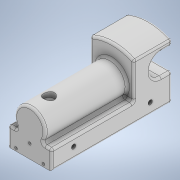
# Autodesk Inventor part: DERKS Train Body
Saved by Autodesk Inventor 2020 (Build 240168000, 168)
## iProperties
Created: 2020-04-30
Part Number: DERKS Train Body
Material: Generic
Document SubType Name: Modeling
Designer: tader
Density: 1 g/cm^3
Appearance: Default
Author: tader
Autodesk Inventor part; units mm, degrees
ref_plane "YZ Plane" through (0, 0, 0) normal (1, 0, 0) x (0, 1, 0)
ref_plane "XZ Plane" through (0, 0, 0) normal (0, 1, 0) x (-1, 0, 0)
ref_plane "XY Plane" through (0, 0, 0) normal (0, 0, 1) x (1, 0, 0)
sketch "Sketch3" plane through (0, 0, 0) normal (1, 0, 0) x (0, 1, 0)
  line L0 (10.0868, 77.2075) -> (-12.1382, 77.2075)
  line L1 (-12.1382, 77.2075) -> (-12.1382, -62.4925)
  line L2 (-12.1382, -62.4925) -> (76.5771, -62.4925)
  line L3 (76.5771, -62.4925) -> (76.5771, -18.0425)
  line L4 (76.5771, -18.0425) -> (10.0868, -18.0425)
  line L5 (10.0868, -18.0425) -> (10.0868, 77.2075)
  point P0 (0, 0)
  dimension "d1" = 22.225
  dimension "d2" = 139.7
  dimension "d3" = 44.45
  constraints: 12 end point, 4 perpendicular, 1 horizontal, 1 vertical
  measures "d1" distance of L0.start L0.end
  measures "d2" distance of L0.end L1.end
  measures "d3" distance of L2.end L3.end
extrude "Extrusion1" add sketch "Sketch3" along normal blind 50.8
sketch "Sketch4" plane through (0, -12.1382, 77.2075) normal (0, 0, 1) x (1, 0, 0)
  line L0 (0, 0) -> (50.8, 0) projected
  line L1 (25.4, 0) -> (25.4, 34.925)
  line L2 (0, 22.225) -> (50.8, 22.225) projected
  arc A0 (37.9356, 22.225) -> (12.8644, 22.225) centre (25.4, 34.925) ccw
  point P0 (0, 12.1382)
  dimension "d6" = 34.925
  constraints: 2 end point, 2 point on circle, 2 point on line, 1 centre point, 1 coincident, 1 midpoint, 1 vertical
  measures "d6" distance of L1.start L1.end
extrude "Extrusion2" add sketch "Sketch4" against normal up to surface (139.7 mm away)
sketch "Sketch5" plane through (50.8, 0, 0) normal (1, 0, 0) x (0, 0, -1)
  line L0 (18.0425, 76.5771) -> (18.0425, 10.0868) projected
  line L1 (18.0425, 76.5771) -> (62.4925, 76.5771)
  line L2 (62.4925, 76.5771) -> (62.4925, 152.7771)
  line L3 (62.4925, 152.7771) -> (18.0425, 152.7771)
  line L4 (18.0425, 152.7771) -> (18.0425, 76.5771)
  point P0 (0, 0)
  dimension "d9" = 76.2
  constraints: 8 end point, 2 parallel, 1 horizontal, 1 perpendicular
  measures "d9" distance of L2.end L1.end
extrude "Extrusion3" add sketch "Sketch5" against normal blind 50.8
sketch "Sketch6" plane through (50.8, 0, 0) normal (1, 0, 0) x (0, 0, -1)
  arc A0 (49.7925, 45.0118) -> (49.7925, 19.6118) centre (49.7925, 32.3118) ccw
  line L0 (62.4925, -12.1382) -> (62.4925, 152.7771) projected
  line L1 (-77.2075, -12.1382) -> (62.4925, -12.1382) projected
  line L2 (49.7925, 45.0118) -> (62.4925, 45.0118)
  line L3 (49.7925, 19.6118) -> (62.4925, 19.6118)
  point P0 (0, 0)
  dimension "d12" = 25.4
  dimension "d13" = 12.7
  dimension "d14" = 44.45
  constraints: 4 end point, 2 perpendicular, 2 point on circle, 2 point on line, 2 tangent, 1 centre point
  measures "d12" diameter of A0
  measures "d13" distance from line of L0 A0.centre
  measures "d14" distance from line of L1 A0.centre
extrude "Extrusion4" cut sketch "Sketch6" against normal blind 50.8
sketch "Sketch7" plane through (50.8, 152.7771, -62.4925) normal (0, 0, -1) x (-1, 0, 0)
  line L0 (0, -107.7653) -> (0, 0) projected
  line L1 (0, -101.4153) -> (50.8, -101.4153)
  arc A0 (50.8, -101.4153) -> (0, -101.4153) centre (25.4, -154.7288) ccw
  line L2 (0, 0) -> (50.8, 0) projected
  line L3 (0, 0) -> (50.8, 0)
  line L4 (50.8, 0) -> (50.8, -101.4153)
  line L5 (0, 0) -> (0, -101.4153)
  point P0 (50.8, -152.7771)
  dimension "d17" = 6.35
  dimension "d18" = 59.055
  constraints: 8 end point, 2 horizontal, 2 point on circle, 1 centre point, 1 collinear, 1 perpendicular, 1 point on line
  measures "d17" distance of L0.start L1.start
  measures "d18" radius of A0
extrude "Extrusion5" cut sketch "Sketch7" against normal blind 50.8 contours L0 L2 L4 A0
sketch "Sketch8" plane through (50.8, 0, 0) normal (1, 0, 0) x (0, 0, -1)
  line L0 (62.4925, -12.1382) -> (62.4925, 19.6118) projected
  line L1 (-77.2075, -12.1382) -> (62.4925, -12.1382) projected
  point P0 (0, 0)
  point P1 (-51.8075, 0.5618)
  point P2 (37.0925, 0.5618)
  dimension "d21" = 25.4
  dimension "d22" = 114.3
  dimension "d23" = 12.7
  dimension "d24" = 12.7
  measures "d21" distance from line of L0 point (37.092, 0.562)
  measures "d22" distance from line of L0 point (-51.808, 0.562)
  measures "d23" distance from line of L1 point (37.092, 0.562)
  measures "d24" distance from line of L1 point (-51.808, 0.562)
hole "Hole1" at (50.8, 0.5618, 51.8075) at (50.8, 0.5618, -37.0925) direction (-1, 0, 0) diameter 4.9784 end through all thread size "1/4-20 UNC" class "2B" standard "ANSI Unified Screw Threads"
sketch "Sketch9" plane through (0, -12.1382, 77.2075) normal (0, 0, 1) x (1, 0, 0)
  circle A0 centre (9.525, 3.175) radius 1.5875
  circle A1 centre (25.4, 15.875) radius 1.5875
  circle A2 centre (41.275, 3.175) radius 1.5875
  line L0 (0, 22.225) -> (0, 0) projected
  line L1 (50.8, 22.225) -> (50.8, 0) projected
  line L2 (0, 0) -> (50.8, 0) projected
  point P0 (0, 12.1382)
  dimension "d32" = 3.175
  dimension "d33" = 3.175
  dimension "d34" = 3.175
  dimension "d35" = 9.525
  dimension "d37" = 25.4
  dimension "d38" = 41.275
  dimension "d39" = 3.175
  dimension "d40" = 3.175
  dimension "d41" = 15.875
  constraints: 3 centre point
  measures "d32" diameter of A0
  measures "d33" diameter of A1
  measures "d34" diameter of A2
  measures "d35" distance from line of L0 A0.centre
  measures "d37" distance from line of L0 A1.centre
  measures "d38" distance from line of L0 A2.centre
  measures "d39" distance from line of L2 A2.centre
  measures "d40" distance from line of L2 A0.centre
  measures "d41" distance from line of L2 A1.centre
extrude "Extrusion6" cut sketch "Sketch9" against normal blind 3.175
sketch "Sketch10" plane through (50.8, -12.1382, -62.4925) normal (0, 0, -1) x (-1, 0, 0)
  circle A0 centre (25.4, 9.525) radius 3.175
  line L0 (50.8, 0) -> (0, 0) projected
  line L1 (50.8, 0) -> (50.8, 31.75) projected
  point P0 (50.8, 12.1382)
  dimension "d44" = 6.35
  dimension "d45" = 9.525
  dimension "d46" = 25.4
  constraints: 1 centre point
  measures "d44" diameter of A0
  measures "d45" distance from line of L0 A0.centre
  measures "d46" distance from line of L1 A0.centre
extrude "Extrusion7" cut sketch "Sketch10" against normal blind 12.7
ref_plane "Work Plane1" through (25.4, 40.6314, 77.2075) normal (0, 1, 0) x (-1, 0, 0)
sketch "Sketch11" plane through (25.4, 40.6314, 77.2075) normal (0, 1, 0) x (-1, 0, 0)
  line L0 (25.4, 0) -> (12.5356, 0) projected
  line L1 (-12.5356, 0) -> (-25.4, 0) projected
  line L2 (17.8446, 0) -> (-17.8446, 0) projected
  line L3 (25.4, -95.25) -> (25.4, 0) projected
  line L4 (-25.4, -95.25) -> (-25.4, 0) projected
  circle A0 centre (0, -22.225) radius 6.35
  point P0 (25.4, -77.2075)
  dimension "d49" = 12.7
  dimension "d50" = 22.225
  constraints: 1 centre point
  measures "d49" diameter of A0
  measures "d50" distance from line of L2 A0.centre
extrude "Extrusion8" cut sketch "Sketch11" against normal blind 6.35
fillet "Fillet2" radius 2.54 32 edges at (0, -1.0257, 77.2075) (6.4322, 10.0868, 77.2075) (25.4, 40.6314, 77.2075) (0, 10.0868, 29.5825) (50.8, 10.0868, 29.5825) (37.9356, 10.0868, 29.5825) (12.8644, 10.0868, 29.5825) (44.3678, 10.0868, 77.2075) (50.8, -1.0257, 77.2075) (50.8, -12.1382, 7.3575) (50.8, 30.7243, -18.0425) (44.3678, 10.0868, -18.0425) (25.4, 40.6314, -18.0425) (25.4, 57.1033, -18.0425) (50.8, 51.3618, -40.2675) (50.8, 45.0118, -56.1425) (50.8, 19.6118, -56.1425) (50.8, 32.3118, -37.0925) (50.8, 3.7368, -62.4925) (25.4, 19.6118, -62.4925) (25.4, 57.1033, -62.4925) (50.8, 48.1868, -62.4925) (0, 48.1868, -62.4925) (25.4, 45.0118, -62.4925) (0, 32.3118, -37.0925) (0, 45.0118, -56.1425) (0, 19.6118, -56.1425) (0, 3.7368, -62.4925) (25.4, -12.1382, -62.4925) (0, 30.7243, -18.0425) (0, 51.3618, -40.2675) (0, -12.1382, 7.3575)
body "Solid1"
